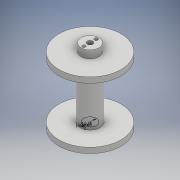
# Autodesk Inventor part: Spool_shaft
Saved by Autodesk Inventor 2017 (Build 210142000, 142)
## iProperties
Created: 2017-04-29
Part Number: Spool_shaft
Material: Generic
Document SubType Name: Modeling
Designer: s4321966
Density: 1 g/cm^3
Appearance: Default
Author: s4321966
Autodesk Inventor part; units mm, degrees
ref_plane "YZ Plane" through (0, 0, 0) normal (1, 0, 0) x (0, 1, 0)
ref_plane "XZ Plane" through (0, 0, 0) normal (0, 1, 0) x (-1, 0, 0)
ref_plane "XY Plane" through (0, 0, 0) normal (0, 0, 1) x (1, 0, 0)
sketch "Sketch1" plane through (0, 0, 0) normal (1, 0, 0) x (0, 1, 0)
  line L0 (0, 0) -> (0, -30)
  line L1 (0, 0) -> (30, 0) construction
  line L2 (0, -30) -> (8, -30)
  line L3 (8, -30) -> (8, -37)
  line L4 (8, -30) -> (15, -30) construction
  line L5 (8, -37) -> (0, -37)
  line L6 (0, -30) -> (0, -32.5)
  line L7 (0, -30) -> (2.5, -30) construction
  line L8 (0, -37) -> (2.5, -37)
  line L9 (0, -37) -> (2.5, -37) construction
  line L10 (2.5, -37) -> (2.5, -76.7172)
  line L11 (2.5, -76.7172) -> (2.5, 69.4116)
  line L12 (8, -30) -> (8, 0)
  line L13 (8, -30) -> (8, -25)
  line L14 (8, -25) -> (28, -25)
  line L15 (28, -25) -> (28, -30)
  line L16 (28, -30) -> (8, -30)
  line L17 (2.5, -37) -> (8, -37)
  line L18 (8, -37) -> (8, 0)
  line L19 (8, 0) -> (2.5, 0)
  line L20 (2.5, 0) -> (2.5, -37)
  line L21 (0, 0) -> (0, 30)
  line L22 (0, 30) -> (8, 30)
  line L23 (8, 30) -> (8, 37)
  line L24 (8, 30) -> (15, 30) construction
  line L25 (8, 37) -> (0, 37)
  line L26 (0, 30) -> (0, 32.5)
  line L27 (0, 30) -> (2.5, 30) construction
  line L28 (0, 37) -> (2.5, 37)
  line L29 (0, 37) -> (2.5, 37) construction
  line L30 (8, 30) -> (8, 0)
  line L31 (8, 30) -> (8, 25)
  line L32 (8, 25) -> (28, 25)
  line L33 (28, 25) -> (28, 30)
  line L34 (28, 30) -> (8, 30)
  line L35 (2.5, 37) -> (8, 37)
  line L36 (8, 37) -> (8, 0)
  line L37 (2.5, 0) -> (2.5, 37)
  line L38 (0, 37) -> (5.75, 37)
  line L39 (8, 25) -> (9, 25)
  line L40 (9, 25) -> (9, -25)
  dimension "d0" = 30
  dimension "d1" = 90
  dimension "d2" = 8
  dimension "d3" = 90
  dimension "d4" = 7
  dimension "d5" = 90
  dimension "d6" = 2.5
  dimension "d7" = 90
  dimension "d8" = 2.5
  dimension "d9" = 0
  dimension "d10" = 5
  dimension "d11" = 20
  dimension "d12" = 90
  dimension "d45" = 5.75
  dimension "d46" = 1
  constraints: 82 end point, 13 symmetric about line, 9 perpendicular, 7 point on line, 6 horizontal, 4 equal length, 2 parallel, 2 vertical, 1 collinear
  measures "d0" distance of L0.start L0.end
  measures "d1" angle of L0 L1
  measures "d2" distance of L0.end L2.end
  measures "d3" angle of L2 L0
  measures "d4" distance of L2.end L3.end
  measures "d5" angle of L3 L4
  measures "d6" distance of L0.end L6.end
  measures "d7" angle of L6 L7
  measures "d8" distance of L5.end L8.end
  measures "d9" distance between parallel lines of L8 L9
  measures "d10" distance of L2.end L13.end
  measures "d11" distance of L13.end L14.end
  measures "d12" angle of L13 L14
  measures "d45" distance of L25.end L38.end
  measures "d46" distance of L31.end L39.end
revolve "Revolution1" add sketch "Sketch1" angle 360 about axis through (0, 0, 0) along (0, 0, -1)
sketch "Sketch3" plane through (0, 0, 0) normal (1, 0, 0) x (0, 1, 0)
  line L0 (0, 0) -> (0, -25)
  line L1 (-28, -25) -> (28, -25) projected
  line L2 (-2.5, -37) -> (2.5, -37) projected
  line L3 (0, -37) -> (0, -13)
  line L4 (0, -13) -> (0, 0)
  line L5 (-54.0631, 0) -> (32.2522, 0)
  circle A0 centre (0, -13) radius 1.5
  line L6 (0, -13) -> (0, -21)
  circle A1 centre (0, -21) radius 1.5
  line L7 (-28, 25) -> (28, 25)
  line L8 (-2.5, 37) -> (2.5, 37)
  line L9 (0, 37) -> (0, 13)
  circle A2 centre (0, 13) radius 1.5
  line L10 (0, 13) -> (0, 21)
  circle A3 centre (0, 21) radius 1.5
  point P0 (0, 25)
  dimension "d14" = 24
  dimension "d15" = 3
  dimension "d16" = 8
  dimension "d17" = 3
  constraints: 18 end point, 10 symmetric about line, 4 centre point, 4 coincident, 3 point on line, 2 midpoint, 1 collinear, 1 horizontal, 2 other
  measures "d14" distance of L3.start L3.end
  measures "d15" diameter of A0
  measures "d16" distance of L6.start L6.end
  measures "d17" diameter of A1
sketch "Sketch4" plane through (0, 0, -37) normal (0, 0, -1) x (-1, 0, 0)
  arc A0 (-1.9966, -1.5104) -> (-1.9966, 1.4896) centre (0.0034, -0.0104) ccw
  line L0 (-1.9966, -0.0104) -> (-1.9966, 1.4896)
  line L1 (-1.9966, -0.0104) -> (-1.9966, -1.5104)
  line L2 (-1.9966, 1.4896) -> (-1.9966, -2.007)
  line L3 (-1.9966, -2.007) -> (-3.9862, -2.007)
  line L4 (-3.9862, -2.007) -> (-3.9862, 1.4896)
  line L5 (-3.9862, 1.4896) -> (-1.9966, 1.4896)
  point P0 (0, 0)
  dimension "d18" = 5
  constraints: 12 end point, 2 parallel, 2 point on circle, 1 centre point, 1 perpendicular, 1 point on line
  measures "d18" diameter of A0
extrude "Extrusion1" add sketch "Sketch4" against normal blind 24 contours L2 L3 L4 L5 L0 L1
extrude "Extrusion2" cut sketch "Sketch3" along normal blind 24 contours A3 L9 | L9 A3 | A2
sketch "Sketch5" plane through (0, 0, -25) normal (0, 0, 1) x (1, 0, 0)
  circle A0 centre (0, 0) radius 8
  circle A1 centre (0, 0) radius 5.625
  circle A2 centre (0, -5.625) radius 1
  circle A3 centre (5.625, 0) radius 1
  circle A4 centre (0, 5.625) radius 1
  circle A5 centre (-5.625, 0) radius 1
  dimension "d23" = 11.25
  dimension "d24" = 2
  dimension "d27" = 360
  constraints: 5 centre point, 2 coincident, 1 vertical alignment, 11 other
  measures "d24" diameter of A2
sketch "Sketch6" plane through (0, 0, -37) normal (0, 0, -1) x (-1, 0, 0)
  circle A0 centre (0, 0) radius 5.5
  circle A1 centre (0, -5.5) radius 1.5
  circle A2 centre (0, 5.5) radius 1.5
  dimension "d29" = 11
  dimension "d30" = 3
  dimension "d33" = 360
  constraints: 2 centre point, 1 coincident, 1 vertical alignment, 7 other
  measures "d30" diameter of A1
extrude "Extrusion3" cut sketch "Sketch6" against normal blind 13 contours A2 A0 | A0 A2 | A1 A0 | A0 A1
sketch "Sketch7" plane through (0, 0, 37) normal (0, 0, 1) x (1, 0, 0)
  circle A0 centre (0, 0) radius 5.5
  circle A1 centre (0, -5.5) radius 1.5
  circle A2 centre (0, 5.5) radius 1.5
  dimension "d37" = 11
  dimension "d38" = 3
  dimension "d41" = 360
  constraints: 2 centre point, 1 coincident, 1 vertical alignment, 7 other
  measures "d38" diameter of A1
extrude "Extrusion4" cut sketch "Sketch7" against normal blind 13 contours A2 A0 | A0 A2 | A1 A0 | A0 A1
body "Solid1"
